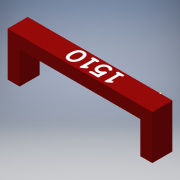
# Autodesk Inventor part: bumper
Saved by Autodesk Inventor 2016 (Build 200138000, 138)
## iProperties
Created: 2016-03-29
Part Number: bumper
Material: Canvas, Blue Stripe
Document SubType Name: Modeling
Designer: gus
Density: 0.152 g/cm^3
Appearance: Red
Author: gus
Autodesk Inventor part; units mm, degrees
ref_plane "YZ Plane" through (0, 0, 0) normal (1, 0, 0) x (0, 1, 0)
ref_plane "XZ Plane" through (0, 0, 0) normal (0, 1, 0) x (-1, 0, 0)
ref_plane "XY Plane" through (0, 0, 0) normal (0, 0, 1) x (1, 0, 0)
sketch "Sketch1" plane through (0, 0, 0) normal (0, 0, 1) x (1, 0, 0)
  line L0 (0, 0) -> (76.2, 0)
  line L1 (76.2, 0) -> (76.2, 279.4)
  line L2 (76.2, 279.4) -> (0, 279.4)
  line L3 (0, 279.4) -> (0, 0)
  line L4 (0, 279.4) -> (-838.2, 279.4)
  line L5 (-838.2, 279.4) -> (-838.2, 203.2)
  line L6 (-838.2, 203.2) -> (0, 203.2)
  line L7 (0, 203.2) -> (0, 279.4)
  line L8 (-838.2, 203.2) -> (-762, 203.2)
  line L9 (-762, 203.2) -> (-762, 0)
  line L10 (-762, 0) -> (-838.2, 0)
  line L11 (-838.2, 0) -> (-838.2, 203.2)
  dimension "d0" = 76.2
  dimension "d1" = 279.4
  dimension "d2" = 838.2
  dimension "d3" = 76.2
  dimension "d4" = 76.2
  dimension "d5" = 203.2
  constraints: 24 end point, 6 parallel, 3 horizontal, 3 perpendicular
  measures "d0" distance of L2.end L1.end
  measures "d1" distance of L1.end L0.end
  measures "d2" distance of L6.end L5.end
  measures "d3" distance of L5.end L4.end
  measures "d4" distance of L9.end L10.end
  measures "d5" distance of L8.end L9.end
extrude "Extrusion1" add sketch "Sketch1" along normal blind 127
sketch "Sketch2" plane through (-838.2, 279.4, 0) normal (0, 1, 0) x (1, 0, 0)
  line L0 (642.6606, -111.4085) -> (325.9156, -111.4085) construction
  line L1 (325.9156, -111.4085) -> (325.9156, -9.0111) construction
  line L2 (325.9156, -9.0111) -> (642.6606, -9.0111) construction
  line L3 (642.6606, -9.0111) -> (642.6606, -111.4085) construction
  point P0 (838.2, 0)
  constraints: 2 other
fillet "Fillet1" radius 25.4 8 edges at (-381, 279.4, 127) (-381, 279.4, 0) (76.2, 139.7, 127) (76.2, 139.7, 0) (76.2, 279.4, 63.5) (-838.2, 279.4, 63.5) (-838.2, 139.7, 127) (-838.2, 139.7, 0)
body "Solid1"
